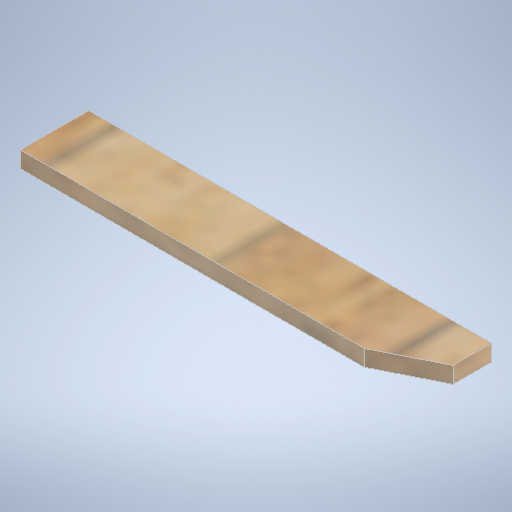
# Autodesk Inventor part: stopper
Saved by Autodesk Inventor 2026.1 (Build 301233020, 233B)
## iProperties
Created: 2025-10-27
Part Number: stopper
Material: 木材 (カエデ材)
Document SubType Name: Modeling
Designer: hibik
Density: 0.67 g/cm^3
Appearance: ナチュラル カエデ材 - 光沢 濃い着色
Author: hibik
Autodesk Inventor part; units mm, degrees
ref_plane "YZ Plane" through (0, 0, 0) normal (1, 0, 0) x (0, 1, 0)
ref_plane "XZ Plane" through (0, 0, 0) normal (0, 1, 0) x (-1, 0, 0)
ref_plane "XY Plane" through (0, 0, 0) normal (0, 0, 1) x (1, 0, 0)
sketch "スケッチ1" plane through (0, 0, 0) normal (0, 1, 0) x (-1, 0, 0)
  line L0 (-68, -11.5) -> (68, -11.5)
  line L1 (68, -11.5) -> (68, 11.5)
  line L2 (68, 11.5) -> (-68, 11.5)
  line L3 (-68, 11.5) -> (-68, -11.5)
  line L4 (-68, -11.5) -> (68, 11.5) construction
  line L5 (68, -11.5) -> (-68, 11.5) construction
  point P0 (0, 0)
  dimension "d0" = 136
  dimension "d1" = 23
  constraints: 12 end point, 2 midpoint, 2 parallel, 1 horizontal, 1 perpendicular
  measures "d0" distance of L1.end L2.end
  measures "d1" distance of L0.end L1.end
extrude "押し出し1" add sketch "スケッチ1" along normal blind 5.5
chamfer "面取り1" distance 20 distance2 10 1 edges at (68, 2.75, 11.5) measured on face at (-22.6667, 3.6667, 11.5)
